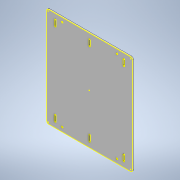
# Autodesk Inventor part: DisplayAcrylicPlate
Saved by Autodesk Inventor 2022 (Build 260153000, 153)
## iProperties
Created: 2021-04-23
Part Number: DisplayAcrylicPlate
Material: Generic
Document SubType Name: Modeling
Designer: Viktor
Density: 1 g/cm^3
Appearance: Default
Author: Viktor
Autodesk Inventor part; units mm, degrees
ref_plane "YZ Plane" through (0, 0, 0) normal (1, 0, 0) x (0, 1, 0)
ref_plane "XZ Plane" through (0, 0, 0) normal (0, 1, 0) x (-1, 0, 0)
ref_plane "XY Plane" through (0, 0, 0) normal (0, 0, 1) x (1, 0, 0)
sketch "Sketch1" plane through (0, 0, 0) normal (0, 0, 1) x (1, 0, 0)
  line L0 (-125, -145) -> (125, -145)
  line L1 (125, -145) -> (125, 145)
  line L2 (125, 145) -> (-125, 145)
  line L3 (-125, 145) -> (-125, -145)
  line L4 (-125, -145) -> (125, 145) construction
  line L5 (125, -145) -> (-125, 145) construction
  point P0 (0, 0)
  dimension "d0" = 250
  dimension "d1" = 290
  constraints: 12 end point, 2 midpoint, 2 parallel, 1 horizontal, 1 perpendicular
  measures "d0" distance of L1.end L2.end
  measures "d1" distance between parallel lines of L0 L2
extrude "Extrusion1" add sketch "Sketch1" along normal blind 3
sketch "Sketch3" plane through (0, 0, 3) normal (0, 0, 1) x (1, 0, 0)
  line L0 (-137.8811, -120.5) -> (156, -120.5) construction
  line L1 (-196.6573, 0) -> (214.7762, 0) construction
  line L2 (-137.8811, 120.5) -> (156, 120.5) construction
  line L3 (-100, -128.5) -> (-100, -112.5) construction
  line L4 (-102.25, -128.5) -> (-102.25, -112.5)
  line L5 (-97.75, -112.5) -> (-97.75, -128.5)
  arc A0 (-102.25, -128.5) -> (-97.75, -128.5) centre (-100, -128.5) ccw
  arc A1 (-97.75, -112.5) -> (-102.25, -112.5) centre (-100, -112.5) ccw
  line L6 (0, -128.5) -> (0, -112.5) construction
  line L7 (2.25, -128.5) -> (2.25, -112.5)
  line L8 (-2.25, -112.5) -> (-2.25, -128.5)
  arc A2 (-2.25, -128.5) -> (2.25, -128.5) centre (0, -128.5) ccw
  arc A3 (2.25, -112.5) -> (-2.25, -112.5) centre (0, -112.5) ccw
  line L9 (0, 203) -> (0, -203) construction
  line L10 (100, -128.5) -> (100, -112.5) construction
  line L11 (102.25, -128.5) -> (102.25, -112.5)
  line L12 (97.75, -112.5) -> (97.75, -128.5)
  arc A4 (97.75, -128.5) -> (102.25, -128.5) centre (100, -128.5) ccw
  arc A5 (102.25, -112.5) -> (97.75, -112.5) centre (100, -112.5) ccw
  line L13 (-100, 128.5) -> (-100, 112.5) construction
  line L14 (-102.25, 128.5) -> (-102.25, 112.5)
  line L15 (-97.75, 112.5) -> (-97.75, 128.5)
  arc A6 (-97.75, 128.5) -> (-102.25, 128.5) centre (-100, 128.5) ccw
  arc A7 (-102.25, 112.5) -> (-97.75, 112.5) centre (-100, 112.5) ccw
  line L16 (0, 128.5) -> (0, 112.5) construction
  line L17 (2.25, 128.5) -> (2.25, 112.5)
  line L18 (-2.25, 112.5) -> (-2.25, 128.5)
  arc A8 (2.25, 128.5) -> (-2.25, 128.5) centre (0, 128.5) ccw
  arc A9 (-2.25, 112.5) -> (2.25, 112.5) centre (0, 112.5) ccw
  arc A10 (97.75, 112.5) -> (102.25, 112.5) centre (100, 112.5) ccw
  line L19 (100, 128.5) -> (100, 112.5) construction
  line L20 (102.25, 128.5) -> (102.25, 112.5)
  line L21 (97.75, 112.5) -> (97.75, 128.5)
  arc A11 (102.25, 128.5) -> (97.75, 128.5) centre (100, 128.5) ccw
  circle A12 centre (-80, -132.5) radius 2.25
  line L22 (-125, -145) -> (125, -145) projected
  circle A13 centre (80, -132.5) radius 2.25
  circle A14 centre (-80, 132.5) radius 2.25
  circle A15 centre (80, 132.5) radius 2.25
  point P0 (0, 0)
  point P1 (-100, -120.5)
  point P2 (0, -120.5)
  point P3 (100, -120.5)
  point P4 (-100, 120.5)
  point P5 (0, 120.5)
  point P6 (100, 120.5)
  dimension "d5" = 16
  dimension "d6" = 16
  dimension "d7" = 2.25
  dimension "d8" = 2.25
  dimension "d9" = 100
  dimension "d10" = 120.5
  dimension "d16" = 80
  dimension "d17" = 12.5
  dimension "d18" = 4.5
  constraints: 52 end point, 33 symmetric about line, 24 point on circle, 16 centre point, 8 tangent, 3 point on line, 2 midpoint, 2 parallel, 2 perpendicular, 1 horizontal, 11 other
  measures "d5" distance of L5.start L5.end
  measures "d6" distance of L7.start L7.end
  measures "d7" radius of A1
  measures "d8" radius of A3
  measures "d9" distance from line of L9 point (-100, -120.5)
  measures "d10" distance of point (0, 0) point (0, -120.5)
  measures "d16" distance from line of L9 A12.centre
  measures "d17" distance from line of L22 A12.centre
  measures "d18" diameter of A12
extrude "Extrusion2" cut sketch "Sketch3" against normal through all
fillet "Fillet1" radius 5 4 edges at (-125, 145, 1.5) (125, 145, 1.5) (125, -145, 1.5) (-125, -145, 1.5)
sketch "Sketch4" plane through (0, 0, 3) normal (0, 0, 1) x (1, 0, 0)
  arc A0 (-125, -140) -> (-120, -145) centre (-120, -140) ccw projected
  line L0 (-120, -145) -> (120, -145) projected
  arc A1 (120, -145) -> (125, -140) centre (120, -140) ccw projected
  line L1 (125, -140) -> (125, 140) projected
  arc A2 (125, 140) -> (120, 145) centre (120, 140) ccw projected
  line L2 (120, 145) -> (-120, 145) projected
  arc A3 (-120, 145) -> (-125, 140) centre (-120, 140) ccw projected
  line L3 (-125, 140) -> (-125, -140) projected
  circle A4 centre (80, -132.5) radius 2.25 projected
  arc A5 (2.25, 128.5) -> (-2.25, 128.5) centre (0, 128.5) ccw projected
  line L4 (2.25, 128.5) -> (2.25, 112.5) projected
  arc A6 (-2.25, 112.5) -> (2.25, 112.5) centre (0, 112.5) ccw projected
  line L5 (-2.25, 112.5) -> (-2.25, 128.5) projected
  arc A7 (97.75, -128.5) -> (102.25, -128.5) centre (100, -128.5) ccw projected
  line L6 (97.75, -128.5) -> (97.75, -112.5) projected
  arc A8 (102.25, -112.5) -> (97.75, -112.5) centre (100, -112.5) ccw projected
  line L7 (102.25, -112.5) -> (102.25, -128.5) projected
  line L8 (-102.25, 112.5) -> (-102.25, 128.5) projected
  arc A9 (-97.75, 128.5) -> (-102.25, 128.5) centre (-100, 128.5) ccw projected
  line L9 (-97.75, 128.5) -> (-97.75, 112.5) projected
  arc A10 (-102.25, 112.5) -> (-97.75, 112.5) centre (-100, 112.5) ccw projected
  circle A11 centre (80, 132.5) radius 2.25 projected
  circle A12 centre (-80, -132.5) radius 2.25 projected
  arc A13 (-102.25, -128.5) -> (-97.75, -128.5) centre (-100, -128.5) ccw projected
  line L10 (-102.25, -128.5) -> (-102.25, -112.5) projected
  arc A14 (-97.75, -112.5) -> (-102.25, -112.5) centre (-100, -112.5) ccw projected
  line L11 (-97.75, -112.5) -> (-97.75, -128.5) projected
  line L12 (-2.25, -128.5) -> (-2.25, -112.5) projected
  arc A15 (2.25, -112.5) -> (-2.25, -112.5) centre (0, -112.5) ccw projected
  line L13 (2.25, -112.5) -> (2.25, -128.5) projected
  arc A16 (-2.25, -128.5) -> (2.25, -128.5) centre (0, -128.5) ccw projected
  arc A17 (97.75, 112.5) -> (102.25, 112.5) centre (100, 112.5) ccw projected
  line L14 (97.75, 112.5) -> (97.75, 128.5) projected
  arc A18 (102.25, 128.5) -> (97.75, 128.5) centre (100, 128.5) ccw projected
  line L15 (102.25, 128.5) -> (102.25, 112.5) projected
  circle A19 centre (-80, 132.5) radius 2.25 projected
  point P0 (0, 0)
equation "\"d6\" = d5"
equation "\"d8\" = d7"
body "Solid1"
